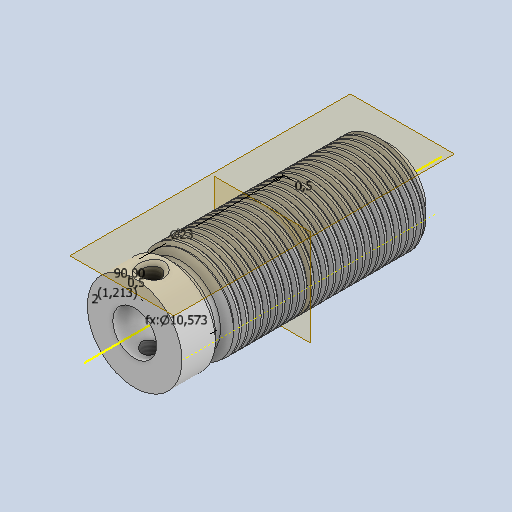
# Autodesk Inventor part: Capston_Drive_Motorwelle
Saved by Autodesk Inventor 2024 (Build 280153000, 153)
## iProperties
Created: 2023-07-19
Part Number: Capston_Drive_Motorwelle
Material: Generisch
Document SubType Name: Modeling
Designer: aewalder
Density: 1 g/cm^3
Appearance: Vorgabe
Pitch: 1,000 mm
Outer_Diameter: 13,000 mm
Author: aewalder
Autodesk Inventor part; units mm, degrees
ref_plane "YZ Plane" through (0, 0, 0) normal (1, 0, 0) x (0, 1, 0)
ref_plane "XY Plane" through (0, 0, 0) normal (0, 0, 1) x (1, 0, 0)
sketch "Sketch1" plane through (0, 0, 0) normal (0, 0, 1) x (1, 0, 0)
  circle A0 centre (0, 0) radius 6.5
  circle A1 centre (0, 0) radius 3
  dimension "d0" = 13
  dimension "d3" = 6
  constraints: 2 centre point, 2 coincident
  measures "d0" diameter of A0
  measures "d3" diameter of A1
extrude "Extrusion1" add sketch "Sketch1" along normal blind 35
sketch "Sketch2" plane through (0, 0, 0) normal (0, 1, 0) x (-1, 0, 0)
  line L0 (-6.5, 0) -> (-6.5, 35) construction
  line L1 (6.5, 0) -> (6.5, 35) projected
  line L2 (6.5, 17.5) -> (-6.5, 17.5) construction
  line L3 (7.0794, 31) -> (5.433, 29.3536)
  line L4 (5.433, 28.6464) -> (7.0794, 27)
  line L5 (7.0794, 27) -> (7.0794, 31)
  line L6 (5.0794, 29) -> (7.0794, 29) construction
  line L7 (7.0794, 4) -> (5.433, 5.6464)
  line L8 (5.433, 6.3536) -> (7.0794, 8)
  line L9 (7.0794, 8) -> (7.0794, 4)
  line L10 (5.0794, 6) -> (7.0794, 6) construction
  line L11 (0, -7) -> (0, 42) projected
  arc A0 (5.433, 29.3536) -> (5.433, 28.6464) centre (5.7866, 29) ccw
  arc A1 (5.433, 6.3536) -> (5.433, 5.6464) centre (5.7866, 6) ccw
  point P0 (0, 0)
  point P1 (6.5, 7.4206)
  point P2 (6.5, 4.5794)
  point P3 (6.5, 27.5794)
  point P4 (6.5, 30.4206)
  point P5 (5.2866, 29)
  dimension "d4" = 90
  dimension "d6" = 2
  dimension "d7" = 23
  dimension "d9" = 0.5
  dimension "d10" = 0.5
  dimension "d34" = 10.5731
  dimension "d35" = 1.2134
  constraints: 18 end point, 5 point on circle, 4 point on line, 4 symmetric about line, 4 tangent, 3 midpoint, 2 centre point, 1 perpendicular, 1 vertical
  measures "d4" angle of L4 L3
  measures "d6" distance from line of L5 L6.start
  measures "d7" diameter of L6 L2
  measures "d9" radius of A0
  measures "d10" radius of A1
  measures "d34" diameter of point (5.287, 29) L11
  measures "d35" distance from line of point (5.287, 29) L1
revolve "Revolution1" cut sketch "Sketch2" angle 360 about axis through (0, 0, -10) along (0, 0, 1) contours L4 A0 L3 L1 | L1 L3 L5 L4
chamfer "Chamfer2" distance 1.5 angle 45 1 edges at (-6.5, 0, 0)
sketch "Sketch3" plane through (0, 0, 0) normal (0, 1, 0) x (-1, 0, 0)
  line L0 (6.5, -0.6458) -> (6.0366, -0.9134)
  line L1 (6.0366, -1.0866) -> (6.5, -1.3542)
  line L2 (6.5, -1.3542) -> (6.5, -0.6458)
  line L3 (5.8866, -1) -> (6.5, -1) construction
  arc A0 (6.0366, -0.9134) -> (6.0366, -1.0866) centre (6.0866, -1) ccw
  line L4 (6.0366, -0.9134) -> (5.8866, -1) construction
  line L5 (5.8866, -1) -> (6.0366, -1.0866) construction
  line L6 (0, -7) -> (0, 42) projected
  line L7 (6.5, 0) -> (6.5, 35) projected
  line L8 (5.0794, 29) -> (7.0794, 29) construction
  point P0 (0, 0)
  dimension "d11" = 60
  dimension "d12" = 0.1
  dimension "d13" = 11.7731
  dimension "d36" = 1
  constraints: 12 end point, 4 tangent, 2 collinear, 2 point on circle, 2 point on line, 1 centre point, 1 equal length, 1 midpoint, 1 vertical
  measures "d11" angle of L1 L0
  measures "d12" radius of A0
  measures "d13" diameter of L3.start L6
  measures "d36" distance from line of L7.start L3
coil "Coil1" sketch "Sketch3" operation cut axis through (0, 0, -10) along (0, 0, 1) pitch 1 turns 30 hand right
ref_plane "Work Plane1" through (0, 6.5, 0) normal (0, 1, 0) x (-1, 0, 0)
sketch "Sketch4" plane through (0, 6.5, 0) normal (0, 1, 0) x (-1, 0, 0)
  line L0 (6.5, 30.4206) -> (-6.5, 30.4206) projected
  line L1 (6.5, 35) -> (-6.5, 35) projected
  line L2 (0, -7) -> (0, 42) projected
  point P0 (0, 0)
  point P1 (0, 32.7103)
  dimension "d22" = 4.5794
  dimension "d23" = 2.2897
  constraints: 1 point on line
  measures "d22" distance between parallel lines of L0 L1
  measures "d23" distance from line of L1 point (0, 32.71)
hole "Hole1" at (0, 6.5, 32.7103) direction (0, -1, 0) diameter 2.459 end through all thread size "M3x0.5" class "6H" standard "ISO Metric profile"
chamfer "Chamfer1" distance 0.5 angle 45 3 edges at (1.2295, 6.3827, 32.712) (-1.2295, 6.3827, 32.7112) (-0.0083, -6.5, 31.4808)
ref_plane "Work Plane2" through (0, 0, 17.5) normal (0, 0, 1) x (1, 0, 0)
equation "\"d0\" = Outer_Diameter"
equation "\"d13\" = d0 - 1.2269 * Pitch"
equation "\"d14\" = Pitch"
equation "\"d23\" = 0.5 * d22"
equation "\"Pitch\" = 1"
equation "\"Outer_Diameter\" = 13"
body "Solid1"
